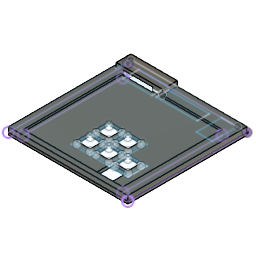
Aiwa up (Autodesk Fusion 360 design; units mm, degrees)
part number: 2026-08-31-21-16-21-827
Autodesk Fusion 360 part; units mm, degrees
sketch "Sketch1" plane through (0, 0, 0) normal (0, 0, 1) x (1, 0, 0)
  line L0 (-50, 42.3306) -> (50, 42.3306)
  line L1 (50, 42.3306) -> (50, -57.6694)
  line L2 (50, -57.6694) -> (-50, -57.6694)
  line L3 (-50, -57.6694) -> (-50, 42.3306)
  line L4 (-60, 57.3306) -> (60, 57.3306)
  line L5 (60, 57.3306) -> (60, -62.6694)
  line L6 (60, -62.6694) -> (-60, -62.6694)
  line L7 (-60, -62.6694) -> (-60, 57.3306)
  dimension "d1" = 120
  dimension "d2" = 120
  dimension "d3" = 5
  dimension "d4" = 10
  dimension "d5" = 10
  dimension "d6" = 15
  constraint horizontal L0
  constraint vertical L1
  constraint horizontal L2
  constraint vertical L3
  constraint horizontal L4
  constraint vertical L5
  constraint horizontal L6
  constraint vertical L7
  measures "d1" distance of L4.start L4.end
  measures "d2" distance of L4.start L6.end
  measures "d3" distance of L2 L6
  measures "d4" distance of L3 L7
  measures "d5" distance of L1 L5
  measures "d6" distance of L0 L4
extrude "Extrude1" add sketch "Sketch1" along normal blind 3 contours L0 L1 L2 L3 makes body 1
extrude "Extrude2" add sketch "Sketch1" along normal blind 5 bodies 1
sketch "Sketch2" plane through (0, 0, 0) normal (0, 0, 1) x (1, 0, 0)
  line L0 (24.775, 54.7196) -> (-16.456, 54.7196)
  line L1 (-16.456, 54.7196) -> (-16.456, 42.3306)
  line L2 (-16.456, 42.3306) -> (24.775, 42.3306)
  line L3 (24.775, 42.3306) -> (24.775, 54.7196)
  line L4 (-60, 57.3306) -> (60, 57.3306)
  line L5 (-60, -62.6694) -> (-60, 57.3306)
  line L6 (60, 57.3306) -> (60, -62.6694)
  line L7 (-20, 57.7123) -> (-49.2058, 57.7123)
  line L8 (-49.2058, 57.7123) -> (-49.2058, 41.7123)
  line L9 (-49.2058, 41.7123) -> (-20, 41.7123)
  line L10 (-20, 41.7123) -> (-20, 57.7123)
  line L11 (50.2041, 57.3306) -> (34.2041, 57.3306)
  line L12 (34.2041, 57.3306) -> (34.2041, 32.0777)
  line L13 (34.2041, 32.0777) -> (50.2041, 32.0777)
  line L14 (50.2041, 32.0777) -> (50.2041, 57.3306)
  line L15 (-50, -57.6694) -> (-50, 42.3306)
  dimension "d11" = 41.231
  dimension "d12" = 12.389
  dimension "d14" = 43.544
  dimension "d15" = 35.225
  dimension "d17" = 16
  dimension "d18" = 16
  dimension "d21" = 29.2058
  dimension "d22" = 0.7942
  constraint horizontal L0
  constraint vertical L1
  constraint horizontal L2
  constraint vertical L3
  constraint horizontal L7
  constraint vertical L8
  constraint horizontal L9
  constraint vertical L10
  constraint horizontal L11
  constraint vertical L12
  constraint horizontal L13
  constraint vertical L14
  constraint coincident L4 L11.start
  measures "d11" distance of L0.start L0.end
  measures "d12" distance of L0.start L2.end
  measures "d14" distance of L1 L5
  measures "d15" distance of L3 L6
  measures "d17" distance of L7 L9
  measures "d18" distance of L11.start L11.end
  measures "d21" distance of L7.start L7.end
  measures "d22" distance of L8 L15
surface "Extrude3" add extruded along (0, 0, 1) between 0 and 1.5 profiles "Sketch2" section 1 contours L4 L11 L12 L13 L14 separate body makes body 2
extrude "Extrude4" cut sketch "Sketch2" along normal blind 2.5 contours L0 L1 L2 L3 bodies 1
sketch "Sketch3" plane through (0, 0, 5) normal (0, 0, 1) x (-1, 0, 0)
  line L0 (-50, 57.6694) -> (50, 57.6694)
  line L1 (50, 57.6694) -> (50, -42.3306)
  line L2 (50, -42.3306) -> (-50, -42.3306)
  line L3 (-50, -42.3306) -> (-50, 57.6694)
  line L4 (60, 62.6694) -> (-60, 62.6694)
  line L5 (-60, 62.6694) -> (-60, -57.3306)
  line L6 (-60, -57.3306) -> (60, -57.3306)
  line L7 (60, -57.3306) -> (60, 62.6694)
  line L8 (56.8458, -57.3306) -> (10.1498, -57.3306)
  line L9 (10.1498, -57.3306) -> (10.1498, -42.3306)
  line L10 (10.1498, -42.3306) -> (56.8458, -42.3306)
  line L11 (56.8458, -42.3306) -> (56.8458, -57.3306)
  constraint horizontal L8
  constraint vertical L9
  constraint horizontal L10
  constraint vertical L11
  constraint coincident L2 L9.end
  constraint coincident L6 L8.start
extrude "Extrude5" add sketch "Sketch3" along normal blind 5 contours L2 L6 L8 L9 L10 L11 bodies 1
extrude "Extrude6" cut sketch "Sketch2" along normal blind 7 contours L4 L8 L9 L10 bodies 1
extrude "Extrude7" add sketch "Sketch1" against normal blind 2.5 separate body makes body 3
extrude "Extrude8" cut sketch "Sketch2" against normal blind 2.5 contours L4 L8 L9 L10 bodies 3
extrude "Extrude9" cut sketch "Sketch2" against normal blind 2.5 contours L0 L1 L2 L3 bodies 3
extrude "Extrude10" cut sketch "Sketch2" against normal blind 2.5 contours L4 L11 L12 L13 L14 bodies 3 makes body 4 at (-56.6667, 12.3306, 0)
sketch "Sketch4" plane through (0, 0, 0) normal (0, 0, 1) x (1, 0, 0)
  line L0 (38, -41.6694) -> (22, -41.6694)
  line L1 (22, -41.6694) -> (22, -56.1694)
  line L2 (22, -56.1694) -> (38, -56.1694)
  line L3 (38, -56.1694) -> (38, -41.6694)
  line L4 (50, -57.6694) -> (-50, -57.6694)
  line L5 (50, 42.3306) -> (50, -57.6694)
  dimension "d37" = 16
  dimension "d38" = 14.5
  dimension "d39" = 1.5
  dimension "d40" = 12
  constraint horizontal L0
  constraint vertical L1
  constraint horizontal L2
  constraint vertical L3
  measures "d37" distance of L0.start L0.end
  measures "d38" distance of L0.start L2.end
  measures "d39" distance of L2 L4
  measures "d40" distance of L3 L5
extrude "Extrude11" cut sketch "Sketch4" along normal blind 3 bodies 1
sketch "Sketch5" plane through (0, 0, 0) normal (0, 0, -1) x (1, 0, 0)
  line L0 (22, 56.1694) -> (38, 56.1694)
  line L1 (38, 56.1694) -> (38, 41.6694)
  line L2 (38, 41.6694) -> (22, 41.6694)
  line L3 (22, 41.6694) -> (22, 56.1694)
  line L4 (-49.2058, -57.3306) -> (-49.2058, -41.7123)
  line L5 (-49.2058, -41.7123) -> (-20, -41.7123)
  line L6 (-20, -41.7123) -> (-20, -57.3306)
  line L7 (-20, -57.3306) -> (60, -57.3306)
  line L8 (60, -57.3306) -> (60, 62.6694)
  line L9 (60, 62.6694) -> (-60, 62.6694)
  line L10 (-60, 62.6694) -> (-60, -57.3306)
  line L11 (-60, -57.3306) -> (-49.2058, -57.3306)
  line L12 (-16.456, -42.3306) -> (24.775, -42.3306)
  line L13 (24.775, -42.3306) -> (24.775, -54.7196)
  line L14 (24.775, -54.7196) -> (-16.456, -54.7196)
  line L15 (-16.456, -54.7196) -> (-16.456, -42.3306)
  line L16 (39, 22.4292) -> (19.95, 22.4292)
  line L17 (19.95, 22.4292) -> (19.95, 41.4792)
  line L18 (19.95, 41.4792) -> (39, 41.4792)
  line L19 (39, 41.4792) -> (39, 22.4292)
  line L20 (50, -42.3306) -> (50, 57.6694)
  line L21 (22.9331, 38.928) -> (35.9331, 38.928)
  line L22 (22.9331, 24.928) -> (35.9331, 24.928)
  line L23 (22.4331, 38.428) -> (22.4331, 25.428)
  line L24 (36.4331, 38.428) -> (36.4331, 25.428)
  arc A0 (22.9331, 38.928) -> (22.4331, 38.428) centre (22.9331, 38.428) ccw
  arc A1 (36.4331, 38.428) -> (35.9331, 38.928) centre (35.9331, 38.428) ccw
  arc A2 (22.4331, 25.428) -> (22.9331, 24.928) centre (22.9331, 25.428) ccw
  arc A3 (35.9331, 24.928) -> (36.4331, 25.428) centre (35.9331, 25.428) ccw
  line L25 (19.9081, 22.403) -> (38.9581, 22.403)
  line L26 (19.9081, 41.453) -> (38.9581, 41.453)
  line L27 (19.9081, 22.403) -> (19.9081, 41.453)
  line L28 (38.9581, 22.403) -> (38.9581, 41.453)
  line L29 (3.9295, 38.9647) -> (16.9295, 38.9647)
  line L30 (3.9295, 24.9647) -> (16.9295, 24.9647)
  line L31 (3.4295, 38.4647) -> (3.4295, 25.4647)
  line L32 (17.4295, 38.4647) -> (17.4295, 25.4647)
  arc A4 (3.9295, 38.9647) -> (3.4295, 38.4647) centre (3.9295, 38.4647) ccw
  arc A5 (17.4295, 38.4647) -> (16.9295, 38.9647) centre (16.9295, 38.4647) ccw
  arc A6 (3.4295, 25.4647) -> (3.9295, 24.9647) centre (3.9295, 25.4647) ccw
  arc A7 (16.9295, 24.9647) -> (17.4295, 25.4647) centre (16.9295, 25.4647) ccw
  line L33 (0.9045, 22.4397) -> (19.9545, 22.4397)
  line L34 (0.9045, 41.4897) -> (19.9545, 41.4897)
  line L35 (0.9045, 22.4397) -> (0.9045, 41.4897)
  line L36 (19.9545, 22.4397) -> (19.9545, 41.4897)
  line L37 (-15.1081, 38.9464) -> (-2.1081, 38.9464)
  line L38 (-15.1081, 24.9464) -> (-2.1081, 24.9464)
  line L39 (-15.6081, 38.4464) -> (-15.6081, 25.4464)
  line L40 (-1.6081, 38.4464) -> (-1.6081, 25.4464)
  arc A8 (-15.1081, 38.9464) -> (-15.6081, 38.4464) centre (-15.1081, 38.4464) ccw
  arc A9 (-1.6081, 38.4464) -> (-2.1081, 38.9464) centre (-2.1081, 38.4464) ccw
  arc A10 (-15.6081, 25.4464) -> (-15.1081, 24.9464) centre (-15.1081, 25.4464) ccw
  arc A11 (-2.1081, 24.9464) -> (-1.6081, 25.4464) centre (-2.1081, 25.4464) ccw
  line L41 (-18.1331, 22.4214) -> (0.9169, 22.4214)
  line L42 (-18.1331, 41.4714) -> (0.9169, 41.4714)
  line L43 (-18.1331, 22.4214) -> (-18.1331, 41.4714)
  line L44 (0.9169, 22.4214) -> (0.9169, 41.4714)
  line L45 (3.9313, 19.8957) -> (16.9313, 19.8957)
  line L46 (3.9313, 5.8957) -> (16.9313, 5.8957)
  line L47 (3.4313, 19.3957) -> (3.4313, 6.3957)
  line L48 (17.4313, 19.3957) -> (17.4313, 6.3957)
  arc A12 (3.9313, 19.8957) -> (3.4313, 19.3957) centre (3.9313, 19.3957) ccw
  arc A13 (17.4313, 19.3957) -> (16.9313, 19.8957) centre (16.9313, 19.3957) ccw
  arc A14 (3.4313, 6.3957) -> (3.9313, 5.8957) centre (3.9313, 6.3957) ccw
  arc A15 (16.9313, 5.8957) -> (17.4313, 6.3957) centre (16.9313, 6.3957) ccw
  line L49 (0.9063, 3.3707) -> (19.9563, 3.3707)
  line L50 (0.9063, 22.4207) -> (19.9563, 22.4207)
  line L51 (0.9063, 3.3707) -> (0.9063, 22.4207)
  line L52 (19.9563, 3.3707) -> (19.9563, 22.4207)
  line L53 (-15.13, 19.904) -> (-2.13, 19.904)
  line L54 (-15.13, 5.904) -> (-2.13, 5.904)
  line L55 (-15.63, 19.404) -> (-15.63, 6.404)
  line L56 (-1.63, 19.404) -> (-1.63, 6.404)
  arc A16 (-15.13, 19.904) -> (-15.63, 19.404) centre (-15.13, 19.404) ccw
  arc A17 (-1.63, 19.404) -> (-2.13, 19.904) centre (-2.13, 19.404) ccw
  arc A18 (-15.63, 6.404) -> (-15.13, 5.904) centre (-15.13, 6.404) ccw
  arc A19 (-2.13, 5.904) -> (-1.63, 6.404) centre (-2.13, 6.404) ccw
  line L57 (-18.155, 3.379) -> (0.895, 3.379)
  line L58 (-18.155, 22.429) -> (0.895, 22.429)
  line L59 (-18.155, 3.379) -> (-18.155, 22.429)
  line L60 (0.895, 3.379) -> (0.895, 22.429)
  dimension "d43" = 19.05
  dimension "d44" = 19.05
  dimension "d45" = 11
  constraint horizontal L16
  constraint vertical L17
  constraint horizontal L18
  constraint vertical L19
  measures "d43" distance of L16.start L16.end
  measures "d44" distance of L16.start L18.end
  measures "d45" distance of L19 L20
extrude "Extrude12" cut sketch "Sketch5" against normal blind 3 contours L21 L22 L23 L24 A0 A1 A2 A3 bodies 1
extrude "Extrude13" cut sketch "Sketch5" against normal blind 3 contours L29 L30 L31 L32 A4 A5 A6 A7 bodies 1
extrude "Extrude14" cut sketch "Sketch5" against normal blind 3 contours L37 L38 L39 L40 A8 A9 A10 A11 bodies 1
extrude "Extrude15" cut sketch "Sketch5" against normal blind 3 contours L53 L54 L55 L56 A16 A17 A18 A19 bodies 1
extrude "Extrude16" cut sketch "Sketch5" against normal blind 3 contours L45 L46 L47 L48 A12 A13 A14 A15 bodies 1
